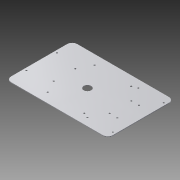
# Autodesk Inventor part: Board 2
Saved by Autodesk Inventor 2015 (Build 190159000, 159)
## iProperties
Created: 2015-05-18
Part Number: Board 2
Material: アルミニウム 6061
Document SubType Name: Modeling
Designer: kenta
Density: 2.7 g/cm^3
Appearance: アルミニウム - フラット - Version 1.1
Mass: 103.87 g
Surface Area: 525.04 cm^2
Volume: 38.4703 cm^3
Author: kenta
Autodesk Inventor part; units mm, degrees
ref_plane "YZ Plane" through (0, 0, 0) normal (1, 0, 0) x (0, 1, 0)
ref_plane "XZ Plane" through (0, 0, 0) normal (0, 1, 0) x (-1, 0, 0)
ref_plane "XY Plane" through (0, 0, 0) normal (0, 0, 1) x (1, 0, 0)
sketch "スケッチ1" plane through (0, 0, 0) normal (0, 0, 1) x (1, 0, 0)
  line L0 (-120, 75) -> (120, 75)
  line L1 (120, 75) -> (120, -75)
  line L2 (120, -75) -> (-120, -75)
  line L3 (-120, -75) -> (-120, 75)
  line L4 (-120, 75) -> (120, -75) construction
  line L5 (120, 75) -> (-120, -75) construction
  point P0 (0, 0)
  dimension "d0" = 240
  dimension "d1" = 150
  constraints: 12 end point, 2 midpoint, 2 parallel, 1 horizontal, 1 perpendicular
  measures "d0" distance of L1.end L2.end
  measures "d1" distance of L0.end L1.end
extrude "押し出し1" add sketch "スケッチ1" along normal blind 1.5
sketch "スケッチ2" plane through (0, 0, 1.5) normal (0, 0, 1) x (1, 0, 0)
  line L0 (-120, 75) -> (-120, -75) projected
  line L1 (120, 75) -> (-120, 75) projected
  line L2 (-120, -75) -> (120, -75) projected
  point P0 (0, 0)
  point P1 (-70, 21.25)
  point P2 (-70, -21.25)
  point P3 (40, 21.25)
  point P4 (40, -21.25)
  point P5 (55, 21.25)
  point P6 (55, -21.25)
  point P7 (-115, 30)
  point P8 (-115, -30)
  dimension "d4" = 50
  dimension "d5" = 53.75
  dimension "d6" = 50
  dimension "d7" = 53.75
  dimension "d8" = 160
  dimension "d9" = 53.75
  dimension "d10" = 53.75
  dimension "d11" = 15
  dimension "d12" = 15
  dimension "d13" = 53.75
  dimension "d14" = 53.75
  dimension "d22" = 60
  dimension "d23" = 30
  dimension "d24" = 5
  dimension "d42" = 42.5
  constraints: 1 vertical alignment
  measures "d4" distance from line of point (-70, 21.25) L0
  measures "d5" distance from line of point (-70, 21.25) L1
  measures "d6" distance from line of point (-70, -21.25) L0
  measures "d7" distance from line of point (-70, -21.25) L2
  measures "d8" distance from line of L0 point (40, 21.25)
  measures "d9" distance from line of point (40, 21.25) L1
  measures "d10" distance from line of L2 point (40, -21.25)
  measures "d11" distance of point (55, 21.25) point (40, 21.25)
  measures "d12" distance of point (55, -21.25) point (40, -21.25)
  measures "d13" distance from line of point (55, 21.25) L1
  measures "d14" distance from line of point (55, -21.25) L2
  measures "d22" distance of point (-115, -30) point (-115, 30)
  measures "d23" vertical distance of point (-115, 30) point (0, 0)
  measures "d24" distance from line of point (-115, 30) L0
  measures "d42" distance of point (-70, -21.25) point (-70, 21.25)
hole "穴1" at (-70, 21.25, 1.5) at (-70, -21.25, 1.5) at (40, 21.25, 1.5) at (40, -21.25, 1.5) at (55, 21.25, 1.5) at (55, -21.25, 1.5) at (-115, 30, 1.5) at (-115, -30, 1.5) direction (0, 0, -1) diameter 3.1 end through all
sketch "スケッチ4" plane through (0, 0, 1.5) normal (0, 0, 1) x (1, 0, 0)
  line L0 (-120, 75) -> (-120, -75) projected
  point P0 (0, 0)
  point P1 (25, 50)
  point P2 (25, -50)
  point P3 (75, 50)
  point P4 (75, -50)
  dimension "d25" = 195
  dimension "d26" = 195
  dimension "d27" = 145
  dimension "d28" = 145
  dimension "d29" = 100
  dimension "d30" = 100
  dimension "d33" = 50
  dimension "d34" = 50
  measures "d25" distance from line of point (75, 50) L0
  measures "d26" distance from line of point (75, -50) L0
  measures "d27" distance from line of point (25, -50) L0
  measures "d28" distance from line of L0 point (25, 50)
  measures "d29" distance of point (25, -50) point (25, 50)
  measures "d30" distance of point (75, -50) point (75, 50)
  measures "d33" vertical distance of point (25, -50) point (0, 0)
  measures "d34" vertical distance of point (0, 0) point (75, -50)
hole "穴2" at (25, 50, 1.5) at (25, -50, 1.5) at (75, 50, 1.5) at (75, -50, 1.5) direction (0, 0, -1) diameter 3.1 depth 3.2 tip angle 118
sketch "スケッチ5" plane through (0, 0, 1.5) normal (0, 0, 1) x (1, 0, 0)
  line L0 (-120, -75) -> (120, -75) projected
  line L1 (120, 75) -> (80, 75)
  line L2 (80, 75) -> (80, -75)
  line L3 (80, -75) -> (120, -75)
  line L4 (120, -75) -> (120, 75)
  point P0 (0, 0)
  dimension "d43" = 40
  constraints: 8 end point, 2 parallel, 1 horizontal, 1 perpendicular, 1 point on line
  measures "d43" distance of L3.end L2.end
extrude "押し出し2" cut sketch "スケッチ5" against normal blind 10
sketch "スケッチ6" plane through (0, 0, 1.5) normal (0, 0, 1) x (1, 0, 0)
  line L0 (-120, -75) -> (80, -75)
  line L1 (80, -75) -> (80, -65)
  line L2 (80, -65) -> (-120, -65)
  line L3 (-120, -65) -> (-120, -75)
  line L4 (-120, 75) -> (80, 75)
  line L5 (80, 75) -> (80, 65)
  line L6 (80, 65) -> (-120, 65)
  line L7 (-120, 65) -> (-120, 75)
  point P0 (0, 0)
  dimension "d46" = 200
  dimension "d47" = 10
  dimension "d48" = 200
  dimension "d49" = 10
  constraints: 16 end point, 4 parallel, 2 horizontal, 2 perpendicular
  measures "d46" distance of L2.end L1.end
  measures "d47" distance of L1.end L0.end
  measures "d48" distance of L5.end L6.end
  measures "d49" distance of L4.end L5.end
extrude "押し出し3" cut sketch "スケッチ6" against normal blind 10
sketch "スケッチ7" plane through (0, 0, 1.5) normal (0, 0, 1) x (1, 0, 0)
  circle A0 centre (-25, 0) radius 7.5
  point P0 (0, 0)
  dimension "d52" = 15
  dimension "d55" = 25
  constraints: 1 centre point
  measures "d52" diameter of A0
  measures "d55" distance of A0.centre point (0, 0)
extrude "押し出し4" cut sketch "スケッチ7" against normal blind 10
fillet "フィレット1" radius 10 4 edges at (80, -65, 0.75) (80, 65, 0.75) (-120, 65, 0.75) (-120, -65, 0.75)
sketch "スケッチ8" plane through (0, 0, 1.5) normal (0, 0, 1) x (1, 0, 0)
  line L0 (-110, -65) -> (70, -65) projected
  line L1 (70, 65) -> (-110, 65) projected
  circle A0 centre (25, 50) radius 1.55 projected
  line L2 (80, -55) -> (80, 55) projected
  point P0 (0, 0)
  point P1 (-57, -46)
  point P2 (15, -46)
  point P3 (-57, 46)
  point P4 (15, 46)
  dimension "d59" = 19
  dimension "d60" = 19
  dimension "d61" = 72
  dimension "d64" = 65
  constraints: 2 horizontal alignment, 2 vertical alignment
  measures "d59" distance from line of point (-57, -46) L0
  measures "d60" distance from line of point (-57, 46) L1
  measures "d61" distance of point (15, -46) point (-57, -46)
  measures "d64" distance from line of point (15, 46) L2
hole "穴3" at (-57, -46, 1.5) at (15, -46, 1.5) at (-57, 46, 1.5) at (15, 46, 1.5) direction (0, 0, -1) diameter 3.2 end through all
